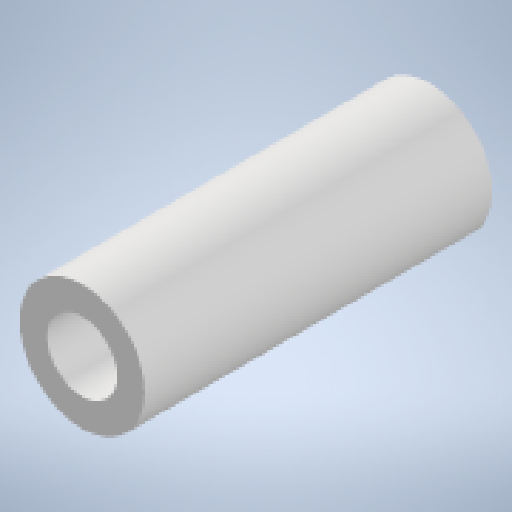
# Autodesk Inventor part: MototMountSpacer
Saved by Autodesk Inventor 2024 (Build 280153020, 153B)
## iProperties
Created: 2024-04-18
Part Number: MototMountSpacer
Material: Generic
Document SubType Name: Modeling
Designer: lvrectanus0
Density: 1 g/cm^3
Appearance: Default
Author: lvrectanus0
Autodesk Inventor part; units mm, degrees
ref_plane "YZ Plane" through (0, 0, 0) normal (1, 0, 0) x (0, 1, 0)
ref_plane "XZ Plane" through (0, 0, 0) normal (0, 1, 0) x (-1, 0, 0)
sketch "Sketch1" plane through (0, 0, 0) normal (0, 0, 1) x (1, 0, 0)
  line L0 (17.7965, -33.0962) -> (17.7965, -30.5346) projected
  arc A0 (25.198, -22.0185) -> (17.7965, -30.5346) centre (26.3965, -30.5346) ccw projected
  arc A1 (3.5113, 31.329) -> (25.198, -22.0185) centre (175.9129, 70.3315) ccw projected
  arc A2 (3.5113, 31.329) -> (-3.5113, 31.329) centre (0, 30.5346) ccw projected
  arc A3 (-25.198, -22.0185) -> (-3.5113, 31.329) centre (-175.9129, 70.3315) ccw projected
  arc A4 (-17.7965, -30.5346) -> (-25.198, -22.0185) centre (-26.3965, -30.5346) ccw projected
  line L1 (-17.7965, -30.5346) -> (-17.7965, -33.0962) projected
  arc A5 (17.7965, -33.0962) -> (-17.7965, -33.0962) centre (0, -209.921) ccw projected
  circle A6 centre (0, 30.5346) radius 2 projected
  circle A7 centre (0, -13.9154) radius 14.2875 projected
  circle A8 centre (0, 30.5346) radius 3.6
  circle A9 centre (0, 30.5346) radius 2
  point P0 (0, 0)
  point P1 (-3.5113, 31.329)
  point P2 (3.5113, 31.329)
  constraints: 2 centre point, 2 coincident, 2 concentric
ref_plane "Work Plane1" through (-29.9965, -34.1346, 20) normal (0, 0, -1) x (0, 1, 0)
extrude "Extrusion1" add sketch "Sketch1" along normal up to surface (20 mm away) contours A8 A2
body "Solid1"
